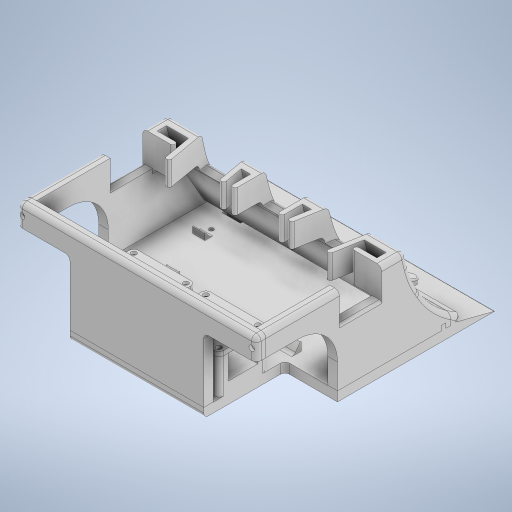
# Autodesk Inventor part: bodyv2
Saved by Autodesk Inventor 2024 (Build 280153000, 153)
## iProperties
Created: 2023-10-20
Part Number: bodyv2
Material: Generic
Document SubType Name: Modeling
Designer: kdcao
Density: 1 g/cm^3
Appearance: Default
Mass: 95.0467 g
Surface Area: 549.579 cm^2
Volume: 95.0467 cm^3
Author: kdcao
Autodesk Inventor part; units mm, degrees
ref_plane "YZ Plane" through (0, 0, 0) normal (1, 0, 0) x (0, 1, 0)
ref_plane "XZ Plane" through (0, 0, 0) normal (0, 1, 0) x (-1, 0, 0)
ref_plane "XY Plane" through (0, 0, 0) normal (0, 0, 1) x (1, 0, 0)
sketch "Sketch1" plane through (0, 0, 0) normal (0, 1, 0) x (-1, 0, 0)
  line L0 (-50, 50) -> (50, 50)
  line L1 (50, 50) -> (50, -50)
  line L2 (50, -50) -> (-50, -50)
  line L3 (-50, -50) -> (-50, 50)
  line L4 (-50, 50) -> (50, -50) construction
  line L5 (50, 50) -> (-50, -50) construction
  point P0 (0, 0)
  dimension "d0" = 100
  dimension "d1" = 100
  constraints: 12 end point, 2 midpoint, 2 parallel, 1 horizontal, 1 perpendicular
  measures "d0" distance of L0.end L1.end
  measures "d1" distance of L1.end L2.end
extrude "Extrusion1" add sketch "Sketch1" along normal blind 40
sketch "Sketch2" plane through (50, 0, 50) normal (1, 0, 0) x (0, 0, -1)
  line L0 (100, 0) -> (100, 40) projected
  line L1 (100, 0.1) -> (76.9136, 8.5028)
  line L2 (76.9136, 8.5028) -> (65.3666, 28.5028)
  line L3 (100, 40) -> (0, 40) projected
  line L4 (100, 40) -> (100, 0.1)
  line L5 (0, 0) -> (100, 0) projected
  line L6 (62.5, 40) -> (65.3666, 28.5028)
  point P0 (50, 0)
  dimension "d4" = 20
  dimension "d5" = 60
  dimension "d6" = 0.1
  dimension "d18" = 62.5
  dimension "d19" = 76
  dimension "d20" = 20
  constraints: 8 end point, 2 point on line, 1 vertical
  measures "d4" angle of L5 L1
  measures "d5" angle of L3 L2
  measures "d6" distance of L0.start L1.start
  measures "d18" distance of L6.start L3.end
  measures "d19" angle of L6 L3
  measures "d20" vertical distance of L1.end L2.end
extrude "Extrusion2" cut sketch "Sketch2" against normal through all
shell "Shell1" thickness 4 removed faces 1 at (16.6667, 40, 29.1667)
sketch "Sketch3" plane through (50, 0, 50) normal (1, 0, 0) x (0, 0, -1)
  circle A0 centre (17.5, 14.5) radius 16.5
  line L0 (0, 0) -> (0, 40) projected
  line L1 (0, 0) -> (100, 0) projected
  line L2 (0, 14.5) -> (0, 0)
  line L3 (0, 0) -> (34, 0)
  line L4 (34, 14.5) -> (34, 0)
  line L5 (17.5, 31) -> (0, 31)
  line L6 (91.2716, 1.5875) -> (0, 1.5875)
  point P0 (50, 0)
  dimension "d12" = 33
  dimension "d13" = 17.5
  dimension "d14" = 14.5
  dimension "d229" = 34
  dimension "d230" = 90
  dimension "d231" = 1.5875
  constraints: 10 end point, 3 point on line, 2 perpendicular, 2 point on circle, 1 centre point, 1 collinear, 1 tangent
  measures "d12" diameter of A0
  measures "d13" distance from line of L0 A0.centre
  measures "d14" distance from line of L1 A0.centre
  measures "d229" distance from line of L0.start L4
  measures "d230" angle of L6 L4
  measures "d231" distance from line of L1 L6.start
extrude "Extrusion3" cut sketch "Sketch3" against normal blind 22 contours A0 L6 | L4 L6 A0 | A0 L6 L0 L5 | L6 L4 L1 A0 | A0 L1 L6 | A0 L1 L0 L6
ref_plane "Work Plane1" through (0, 0, -50) normal (1, 0, 0) x (0, 0, -1)
mirror "Mirror1" about plane through (0, 0, -50) normal (1, 0, 0) of "Extrusion3"
fillet "Fillet1" radius 43.275 1 edges at (0, 8.5028, -26.9136)
fillet "Fillet2" radius 40 1 edges at (0, 28.5028, -15.3666)
sketch "Sketch27" plane through (-50, 40, 50) normal (0, 0, 1) x (1, 0, 0)
  line L0 (0, -9) -> (0, 0) projected
  line L1 (100, -9) -> (100, 0) projected
  point P0 (50, -40)
  point P1 (2, -4.5)
  point P2 (98, -4.5)
  point P3 (0, -4.5)
  point P4 (100, -4.5)
  dimension "d156" = 2
  dimension "d157" = 0
  dimension "d158" = 2
  dimension "d159" = 0
  constraints: 2 midpoint
  measures "d156" distance from line of L0 point (2, -4.5)
  measures "d157" vertical distance of point (0, -4.5) point (2, -4.5)
  measures "d158" distance from line of L1 point (98, -4.5)
  measures "d159" vertical distance of point (100, -4.5) point (98, -4.5)
hole "Hole5" at (-48, 35.5, 50) at (48, 35.5, 50) direction (0, 0, -1) diameter 1.75 depth 5.83 counterbore diameter 2.2 counterbore depth 1.2
sketch "Sketch28" plane through (0, 0, 0) normal (0, -1, 0) x (1, 0, 0)
  line L0 (-28, 50) -> (28, 50) projected
  line L1 (28, 16) -> (28, 50) projected
  line L2 (-28, 50) -> (-28, 16) projected
  line L3 (-50, -50) -> (-50, 16) projected
  line L4 (-28, 16) -> (-50, 16) projected
  line L5 (50, 16) -> (28, 16) projected
  line L6 (50, 16) -> (50, -50) projected
  point P0 (0, 0)
  point P1 (-24, 48)
  point P2 (24, 48)
  point P3 (-48, 12)
  point P4 (48, 12)
  dimension "d160" = 2
  dimension "d161" = 2
  dimension "d162" = 4
  dimension "d163" = 4
  dimension "d164" = 2
  dimension "d165" = 4
  dimension "d166" = 4
  dimension "d167" = 2
  measures "d160" distance from line of L0 point (-24, 48)
  measures "d161" distance from line of L0 point (24, 48)
  measures "d162" distance from line of L1 point (24, 48)
  measures "d163" distance from line of L2 point (-24, 48)
  measures "d164" distance from line of L3 point (-48, 12)
  measures "d165" distance from line of L4 point (-48, 12)
  measures "d166" distance from line of L5 point (48, 12)
  measures "d167" distance from line of L6 point (48, 12)
hole "Hole6" at (-24, 0, 48) at (24, 0, 48) at (-48, 0, 12) at (48, 0, 12) direction (0, 1, 0) diameter 1.75 depth 5.83 counterbore diameter 2.2 counterbore depth 1.2
sketch "Sketch4" plane through (50, 40, 50) normal (1, 0, 0) x (0, 0, -1)
  line L0 (-2.2168, -36) -> (77.4409, -36)
  arc A0 (69.0382, -17.8566) -> (91.7145, -36.8843) centre (106.5154, 3.7809) ccw projected
  line L1 (34, -40) -> (100, -40) projected
  line L2 (77.4409, -36) -> (77.4409, -34)
  line L3 (77.4409, -34) -> (79.4409, -34)
  line L4 (79.4409, -36) -> (81.4409, -36)
  line L5 (78.6988, -29.3469) -> (78.6988, -29.3697)
  line L6 (79.4409, -34) -> (79.4409, -36)
  line L7 (81.4409, -36) -> (81.4409, -31.4894)
  line L8 (0, -40) -> (0, -9) projected
  point P0 (50, -40)
  point P1 (78.6988, -29.3697)
  dimension "d73" = 2
  dimension "d75" = 4
  dimension "d76" = 2
  dimension "d77" = 2
  dimension "d78" = 2
  dimension "d79" = 81.4409
  constraints: 14 end point, 3 perpendicular, 3 point on circle, 2 vertical, 1 horizontal
  measures "d73" distance of L2.end L3.end
  measures "d75" distance between parallel lines of L1 L0
  measures "d76" distance of L0.end L2.end
  measures "d77" distance of L3.end L4.start
  measures "d78" distance of L4.start L4.end
  measures "d79" distance from line of L8 L4.end
split body "Split1" sketch "Sketch4" result two bodies curves L0 L2 L3 L6 L4 L7 first body at (9.3333, 22, 49.5)
sketch "Sketch5" plane through (-50, 0, -50) normal (-1, 0, 0) x (0, 0, 1)
  line L0 (66, 4) -> (22.5591, 4) projected
  line L1 (39.2, 4) -> (39.2, 7)
  line L2 (39.2, 7) -> (36.8561, 4)
  line L3 (36.8561, 4) -> (39.2, 4)
  line L4 (100, 4) -> (100, 0) projected
  line L5 (66, 0) -> (66, 4) projected
  point P0 (50, 0)
  point P1 (17.4103, 4)
  dimension "d28" = 3
  dimension "d29" = 38
  dimension "d43" = 26.8
  constraints: 6 end point, 2 perpendicular, 1 point on line
  measures "d28" distance of L1.start L1.end
  measures "d29" angle of L1 L2
  measures "d43" distance from line of L1.start L5
ref_plane "Work Plane2" through (-37.5, 0, -50) normal (-1, 0, 0) x (0, 0, 1)
extrude "Extrusion4" add sketch "Sketch5" against normal blind 5.15 from surface at -12.5 bodies 3
sketch "Sketch6" plane through (-28, 0, 16) normal (-1, 0, 0) x (0, 0, 1)
  line L0 (34, 4) -> (0, 4) projected
  line L1 (7.3, 4) -> (7.3, 18.6)
  line L2 (7.3, 18.6) -> (11.3, 18.6)
  line L3 (11.3, 18.6) -> (11.3, 8.5)
  line L4 (11.3, 8.5) -> (23.7, 8.5)
  line L5 (23.7, 8.5) -> (23.7, 18.6)
  line L6 (23.7, 18.6) -> (27.7, 18.6)
  line L7 (27.7, 18.6) -> (27.7, 4)
  line L8 (7.3, 4) -> (27.7, 4)
  line L9 (34, 4) -> (34, 0) projected
  line L10 (7.3, 18.6) -> (27.7, 18.6)
  line L11 (27.7, 18.6) -> (27.7, 20.6)
  line L12 (27.7, 20.6) -> (7.3, 20.6)
  line L13 (7.3, 20.6) -> (7.3, 18.6)
  point P0 (-16, 0)
  point P1 (27.7, 18.6)
  dimension "d34" = 12.4
  dimension "d38" = 4
  dimension "d39" = 4
  dimension "d40" = 10.3
  dimension "d168" = 10.1
  dimension "d169" = 14.6
  dimension "d170" = 2
  dimension "d171" = 20.4
  constraints: 24 end point, 7 perpendicular, 4 point on line, 2 parallel, 1 collinear, 1 horizontal
  measures "d34" distance of L3.end L4.end
  measures "d38" distance of L5.end L6.end
  measures "d39" distance of L1.end L2.end
  measures "d40" distance between parallel lines of L9 L5
  measures "d168" distance of L2.end L3.end
  measures "d169" distance of L6.end L7.end
  measures "d170" distance of L12.end L1.end
  measures "d171" distance of L11.end L12.end
extrude "Extrusion5" add sketch "Sketch6" against normal blind 25.7875 contours L0 L1 L2 L3 L4 L5 L6 L7 | L6 L10 L2 L13 L12 L11 bodies 3
mirror "Mirror2" about plane through (0, 0, -50) normal (1, 0, 0) of "Extrusion5", "Extrusion4" bodies 3
sketch "Sketch7" plane through (-28, 0, 16) normal (-1, 0, 0) x (0, 0, 1)
  line L0 (-6.8, 4) -> (-6.8, 8)
  line L1 (-6.8, 8) -> (-3.8, 4)
  line L2 (-26.8, 7) -> (-26.8, 4) projected
  line L3 (-6.8, 4) -> (-3.8, 4)
  point P0 (-16, 0)
  point P1 (0, 4)
  dimension "d45" = 3
  dimension "d46" = 4
  dimension "d232" = 20
  constraints: 6 end point, 1 horizontal, 1 point on line
  measures "d45" distance from line of L1.end L0
  measures "d46" distance of L0.start L0.end
  measures "d232" distance between parallel lines of L0 L2
extrude "Extrusion6" add sketch "Sketch7" against normal blind 5.15 bodies 3
mirror "Mirror3" about plane through (0, 0, -50) normal (1, 0, 0) of "Extrusion6" bodies 3
sketch "Sketch9" plane through (28, 4, 16) normal (0, 1, 0) x (1, 0, 0)
  line L0 (-66.85, 42.8) -> (-59.15, 42.8)
  line L1 (-59.15, 42.8) -> (-59.15, 30)
  line L2 (-59.15, 30) -> (-66.85, 30)
  line L3 (-66.85, 30) -> (-66.85, 42.8)
  line L4 (-66.85, 42.8) -> (-59.15, 30) construction
  line L5 (-59.15, 42.8) -> (-66.85, 30) construction
  line L6 (-78, 0) -> (-78, 43.4409) projected
  line L7 (-78, 0) -> (-56, 0) projected
  point P0 (-28, 16)
  point P1 (-63, 36.4)
  point P2 (-78, 48.5897)
  point P3 (-63, 30)
  dimension "d49" = 12.8
  dimension "d50" = 7.7
  dimension "d51" = 15
  dimension "d52" = 30
  constraints: 12 end point, 3 midpoint, 2 parallel, 1 horizontal, 1 perpendicular
  measures "d49" distance of L2.end L0.start
  measures "d50" distance of L1.end L2.end
  measures "d51" distance from line of L6 point (-63, 30)
  measures "d52" distance between parallel lines of L7 L2
extrude "Extrusion7" cut sketch "Sketch9" along normal blind 3 from surface at -4 bodies 3
mirror "Mirror4" about plane through (0, 0, -50) normal (1, 0, 0) of "Extrusion7" bodies 3
ref_plane "Work Plane4" through (-50, 40, -10.5) normal (0, 0, 1) x (1, 0, 0)
sketch "Sketch12" plane through (-50, 40, -10.5) normal (0, 0, 1) x (1, 0, 0)
  line L0 (50.0586, -12.0127) -> (41.2086, -12.0127)
  line L1 (41.2086, -12.0127) -> (41.2086, 0.5873)
  line L2 (41.2086, 0.5873) -> (58.9086, 0.5873)
  line L3 (58.9086, 0.5873) -> (58.9086, -12.0127)
  line L4 (58.9086, -12.0127) -> (50.0586, -12.0127)
  point P0 (50, -40)
  dimension "d61" = 12.6
  dimension "d62" = 17.7
  constraints: 10 end point, 4 perpendicular, 1 collinear, 1 horizontal, 1 point on line
  measures "d61" distance of L2.end L3.end
  measures "d62" distance of L1.end L2.end
extrude "Extrusion9" cut sketch "Sketch12" along normal mid plane 14.7625 bodies 2
ref_plane "Work Plane5" through (34.4281, 50.6, -7.4264) normal (0.1736482, 0, -0.9848078) x (0, -1, 0)
sketch "Sketch13" plane through (34.4281, 50.6, -7.4264) normal (0.1736482, 0, -0.9848078) x (0, -1, 0)
  line L0 (10.6, -0.1431) -> (23.2, -0.1431)
  line L1 (23.2, -0.1431) -> (23.2, 17.5569)
  line L2 (23.2, 17.5569) -> (10.6, 17.5569)
  line L3 (10.6, 17.5569) -> (10.6, -0.1431)
  line L4 (10.6, 25.2969) -> (10.6, -11.231) projected
  line L5 (10.6, 25.2969) -> (22.6127, 25.817) projected
  point P0 (50.6, 32.6154)
  point P1 (16.6063, 25.5569)
  dimension "d65" = 17.7
  dimension "d66" = 12.6
  dimension "d263" = 8
  constraints: 8 end point, 2 parallel, 1 horizontal, 1 midpoint, 1 perpendicular, 1 point on line
  measures "d65" distance of L2.end L0.start
  measures "d66" distance of L1.end L2.end
  measures "d263" distance from line of point (16.606, 25.557) L2
extrude "Extrusion10" cut sketch "Sketch13" along normal mid plane 20 bodies 2
ref_plane "Work Plane6" through (-34.4281, 38, -7.4264) normal (0.1736482, 0, 0.9848078) x (0, 1, 0)
sketch "Sketch14" plane through (-34.4281, 38, -7.4264) normal (0.1736482, 0, 0.9848078) x (0, 1, 0)
  line L0 (-10.6, -0.8394) -> (2, -0.8394)
  line L1 (2, -0.8394) -> (2, -17.4394)
  line L2 (2, -17.4394) -> (-10.6, -17.4394)
  line L3 (-10.6, -17.4394) -> (-10.6, -0.8394)
  line L4 (2, 11.231) -> (2, -25.4124) projected
  line L5 (-10.0127, -25.9325) -> (2, -25.4124) projected
  point P0 (-38, -32.6154)
  point P1 (-4.0063, -25.6724)
  dimension "d69" = 16.6
  dimension "d70" = 12.6
  constraints: 8 end point, 2 parallel, 1 horizontal, 1 midpoint, 1 perpendicular, 1 point on line
  measures "d69" distance of L0.end L1.end
  measures "d70" distance of L1.end L2.end
extrude "Extrusion11" cut sketch "Sketch14" along normal mid plane 20 bodies 2
sketch "Sketch15" plane through (0, 0, 0) normal (0, -1, 0) x (1, 0, 0)
  line L0 (31.15, -26.8) -> (31.15, -14) projected
  line L1 (38.85, -26.8) -> (31.15, -26.8) projected
  line L2 (31.15, -24.5) -> (38.85, -24.5)
  line L3 (38.85, -24.5) -> (38.85, -26.8)
  line L4 (38.85, -26.8) -> (31.15, -26.8)
  line L5 (31.15, -26.8) -> (31.15, -24.5)
  circle A0 centre (35, -16.1508) radius 0.875
  line L6 (50, 16) -> (50, -50) projected
  line L7 (50, -50) -> (-50, -50) projected
  point P0 (0, 0)
  dimension "d80" = 15
  dimension "d81" = 1.75
  dimension "d82" = 2.3
  dimension "d83" = 33.8492
  constraints: 8 end point, 2 parallel, 1 centre point, 1 horizontal, 1 perpendicular, 1 point on line
  measures "d80" distance from line of L6 A0.centre
  measures "d81" diameter of A0
  measures "d82" distance of L2.end L1.start
  measures "d83" distance from line of L7 A0.centre
extrude "Extrusion12" cut sketch "Sketch15" against normal through all bodies 3
mirror "Mirror5" about plane through (0, 0, -50) normal (1, 0, 0) of "Extrusion12" bodies 3
sketch "Sketch16" plane through (50, 40, 50) normal (1, 0, 0) x (0, 0, -1)
  line L0 (4, -20.7805) -> (4, 0)
  line L1 (0, -9) -> (0, 0) projected
  point P0 (50, -40)
  dimension "d86" = 4
  constraints: 2 end point
  measures "d86" distance between parallel lines of L1 L0
split body "Split2" sketch "Sketch16" result two bodies bodies 2 curves L0 first body at (9.3333, 22, 49.5)
sketch "Sketch17" plane through (0, 40, 0) normal (0, 1, 0) x (1, 0, 0)
  line L0 (35.4679, 12.5) -> (32.6467, -3.5)
  line L1 (32.6467, -3.5) -> (34.6467, -3.8527)
  line L2 (34.6467, -3.8527) -> (37.4679, 12.1473)
  line L3 (37.4679, 12.1473) -> (35.4679, 12.5)
  line L4 (17.4949, 12.5) -> (15.2026, -0.5)
  line L5 (15.2026, -0.5) -> (13.2026, -0.1473)
  line L6 (13.2026, -0.1473) -> (15.4327, 12.5)
  line L7 (16.768, 8.3776) -> (17.4949, 12.5) projected
  line L8 (17.4949, 12.5) -> (8.9086, 12.5) projected
  line L9 (15.4327, 12.5) -> (17.4949, 12.5)
  point P0 (0, 0)
  point P1 (17.1314, 10.4388)
  point P2 (14.2026, -0.3237)
  dimension "d87" = 2
  dimension "d88" = 16
  dimension "d89" = 2
  dimension "d264" = 17.7
  dimension "d266" = 13
  constraints: 16 end point, 4 parallel, 2 midpoint, 2 perpendicular, 1 horizontal
  measures "d87" horizontal distance of L0.end L1.end
  measures "d88" vertical distance of L1.end L2.end
  measures "d89" horizontal distance of L4.end L5.end
  measures "d264" distance from line of point (17.131, 10.439) L0
  measures "d266" vertical distance of L4.start L4.end
extrude "Extrusion13" add sketch "Sketch17" against normal blind 10 bodies 5
mirror "Mirror6" about plane through (0, 0, -50) normal (1, 0, 0) of "Extrusion13" bodies 5
sketch "Sketch18" plane through (0, 40, 0) normal (0, 1, 0) x (1, 0, 0)
  line L0 (17.4949, 12.5) -> (8.9086, 12.5) projected
  line L1 (8.9086, 12.5) -> (8.9086, 0)
  line L2 (8.9086, 0) -> (10.9086, 0)
  line L3 (10.9086, 0) -> (10.9086, 12.5)
  line L4 (10.9086, 12.5) -> (8.9086, 12.5)
  line L5 (-8.7914, 16.0057) -> (-8.7914, 11.3726) projected
  line L6 (-8.7914, 12.5) -> (-8.7914, 0)
  line L7 (-8.7914, 0) -> (-10.7914, 0)
  line L8 (-10.7914, 0) -> (-10.7914, 12.5)
  line L9 (-10.7914, 12.5) -> (-8.7914, 12.5)
  point P0 (0, 0)
  point P1 (-8.7914, 15.4951)
  point P2 (-8.7914, 11.3726)
  dimension "d94" = 2
  dimension "d95" = 2
  dimension "d96" = 12.5
  constraints: 16 end point, 4 parallel, 3 perpendicular, 3 point on line, 1 collinear
  measures "d94" distance of L1.end L2.end
  measures "d95" distance of L6.end L7.end
  measures "d96" distance of L2.end L3.end
extrude "Extrusion14" add sketch "Sketch18" against normal blind 10 bodies 5
sketch "Sketch31" plane through (-28, 20.6, 43.7) normal (0, 1, 0) x (1, 0, 0)
  line L0 (0, 20.4) -> (25.7875, 20.4) projected
  line L1 (25.7875, 20.4) -> (25.7875, 0) projected
  line L2 (0, 0) -> (25.7875, 0) projected
  line L3 (0, 0) -> (0, 20.4) projected
  point P0 (28, 43.7)
  point P1 (23.7875, 18.4)
  point P2 (23.7875, 2)
  point P3 (2, 2)
  point P4 (2, 18.4)
  dimension "d180" = 2
  dimension "d181" = 2
  dimension "d182" = 2
  dimension "d183" = 2
  dimension "d184" = 2
  dimension "d185" = 2
  dimension "d186" = 2
  dimension "d187" = 2
  measures "d180" distance from line of L0 point (23.787, 18.4)
  measures "d181" distance from line of L1 point (23.787, 18.4)
  measures "d182" distance from line of L1 point (23.787, 2)
  measures "d183" distance from line of L2 point (23.787, 2)
  measures "d184" distance from line of L2 point (2, 2)
  measures "d185" distance from line of L3 point (2, 2)
  measures "d186" distance from line of L0 point (2, 18.4)
  measures "d187" distance from line of L3 point (2, 18.4)
hole "Hole7" at (-4.2125, 20.6, 25.3) at (-4.2125, 20.6, 41.7) at (-26, 20.6, 41.7) at (-26, 20.6, 25.3) direction (0, -1, 0) diameter 1.75 depth 5.83 counterbore diameter 2.2 counterbore depth 1.2 bodies 3
mirror "Mirror7" about plane through (0, 0, -50) normal (1, 0, 0) of "Hole7" bodies 3
sketch "Sketch32" plane through (-28, 0, 16) normal (-1, 0, 0) x (0, 0, 1)
  line L0 (7.3, 4) -> (7.3, 20.6) projected
  line L1 (7.3, 18.6) -> (27.7, 18.6)
  line L2 (27.7, 20.6) -> (27.7, 4) projected
  point P0 (-16, 0)
  point P1 (11.3, 18.6)
  constraints: 3 point on line, 2 end point, 1 horizontal
split body "Split6" sketch "Sketch32" result two bodies bodies 3 curves L1 first body at (11.7768, 20.1, 36.025) (-11.7768, 20.1, 36.025)
fillet "Fillet4" radius 2 8 edges at (-28, 19.6, 43.7) (-28, 19.6, 23.3) (-2.2125, 19.6, 23.3) (-2.2125, 19.6, 43.7) (-28, 11.3, 43.7) (-28, 11.3, 23.3) (-2.2125, 11.3, 23.3) (-2.2125, 11.3, 43.7)
mirror "Mirror8" about plane through (0, 0, -50) normal (1, 0, 0) of "Fillet4"
sketch "Sketch34" plane through (0, 40, 0) normal (0, 1, 0) x (1, 0, 0)
  line L0 (-46, -46) -> (-46, 8.3776) projected
  line L1 (-50, -32.5) -> (-50, -16) projected
  line L2 (-46, 2.5) -> (-50, 2.5)
  line L3 (-50, 2.5) -> (-50, -15.2)
  line L4 (-50, -15.2) -> (-46, -15.2)
  line L5 (-46, -15.2) -> (-46, 2.5)
  line L6 (-34.4703, 12.5) -> (-50, 12.5) projected
  point P0 (0, 0)
  point P1 (-46, -15.2)
  dimension "d196" = 17.7
  dimension "d197" = 10
  constraints: 8 end point, 2 parallel, 2 point on line, 1 horizontal, 1 perpendicular
  measures "d196" distance of L2.end L3.end
  measures "d197" distance between parallel lines of L6 L2
extrude "Extrusion15" cut sketch "Sketch34" against normal blind 12.6 bodies 5
sketch "Sketch35" plane through (0, 40, 0) normal (0, 1, 0) x (1, 0, 0)
  line L0 (-50, 12.5) -> (-50, 2.5) projected
  line L1 (-50, 2.5) -> (-37.5, 2.5)
  line L2 (-37.5, 2.5) -> (-37.5, 4.5)
  line L3 (-37.5, 4.5) -> (-50, 4.5)
  line L4 (-50, 4.5) -> (-50, 2.5)
  point P0 (0, 0)
  dimension "d200" = 12.5
  dimension "d201" = 2
  constraints: 8 end point, 2 parallel, 1 horizontal, 1 perpendicular
  measures "d200" distance of L2.end L3.end
  measures "d201" distance of L1.end L2.end
extrude "Extrusion16" add sketch "Sketch35" against normal blind 12.6 bodies 5
mirror "Mirror9" about plane through (0, 0, -50) normal (1, 0, 0) of "Extrusion15", "Extrusion16" bodies 5
fillet "Fillet8" radius 2 26 edges at (50, 40, 48) (0, 40, 50) (-50, 40, 48) (50, 35.5, 50) (-50, 35.5, 50) (-28, 31, 48) (28, 31, 48) (50, 40, -7.5) (42.734, 40, -12.5) (50, 40, 30.6) (-50, 40, 30.6) (-50, 40, -7.5) (-42.2351, 40, -12.5) (-13.2028, 40, -12.5) (13.2018, 40, -12.5) (50, 22.8888, -18.6078) (50, 14.659, -24.5054) (50, 36.9787, -13.2533) (50, 28.65, -15.7311) (-50, 22.8888, -18.6078) (-50, 28.65, -15.7311) (-50, 36.9787, -13.2533) (-50, 14.659, -24.5054) (0, 0, 50) (28, 2, 16) (-28, 2, 16)
fillet "Fillet9" radius 1 18 edges at (-50, 27.4, 6.35) (50, 27.4, 6.35) (37.5, 33.7, -4.5) (37.5, 33.7, -2.5) (32.6467, 35, 3.5) (34.6467, 35, 3.8527) (13.2026, 35, 0.1473) (15.2026, 35, 0.5) (10.9086, 35, 0) (8.9086, 35, 0) (-8.7914, 35, 0) (-10.7914, 35, 0) (-15.2026, 35, 0.5) (-13.2026, 35, 0.1473) (-32.6467, 35, 3.5) (-34.6467, 35, 3.8527) (-37.5, 33.7, -4.5) (-37.5, 33.7, -2.5)
sketch "Sketch36" plane through (-50, 0, -50) normal (-1, 0, 0) x (0, 0, 1)
  arc A0 (8.2855, 3.1157) -> (18.5591, 8.5106) centre (-6.5154, 43.7809) ccw projected
  line L0 (18.5591, 4) -> (18.5591, 8.5106) projected
  line L1 (0, 0) -> (66, 0) projected
  line L2 (0.15, 0) -> (14.55, 3.6975)
  line L3 (14.55, 3.6975) -> (14.0365, 5.6975)
  line L4 (14.0365, 5.6975) -> (-1.9913, 0)
  line L5 (-1.9913, 0) -> (0.15, 0)
  line L6 (0.2518, 0.0261) -> (0.4, 0)
  line L7 (0.15, 0) -> (0.4, 0)
  point P0 (50, 0)
  dimension "d210" = 2
  dimension "d211" = 0.15
  dimension "d213" = 14.4
  dimension "d214" = 17.0103
  dimension "d226" = 0.25
  dimension "d227" = 10
  constraints: 12 end point, 4 point on line, 1 collinear, 1 horizontal, 1 perpendicular, 1 point on circle
  measures "d210" vertical distance of L2.end L3.end
  measures "d211" distance of L1.start L2.start
  measures "d213" horizontal distance of L2.end L2.start
  measures "d214" distance of L3.end L4.end
  measures "d226" distance of L2.start L6.end
  measures "d227" angle of L1 L6
extrude "Extrusion17" cut sketch "Sketch36" against normal through all bodies 7
sketch "Sketch37" plane through (-50, 0, -49.85) normal (0, 0.9685803, -0.2487012) x (1, 0, 0)
  circle A0 centre (26, -10.1171) radius 2.5
  line L0 (0, -14.8671) -> (0, -0.1051) projected
  line L1 (100, -14.8671) -> (0, -14.8671) projected
  point P0 (50, -48.2837)
  point P1 (0, 0)
  dimension "d217" = 5
  dimension "d218" = 26
  dimension "d219" = 4.75
  constraints: 1 centre point
  measures "d217" diameter of A0
  measures "d218" distance from line of L0 A0.centre
  measures "d219" distance from line of L1 A0.centre
extrude "Extrusion18" add sketch "Sketch37" along normal blind 2 bodies 7
fillet "Fillet10" radius 0.5 1 edges at (-26.5, 4.4533, -40.5482)
mirror "Mirror10" about plane through (0, 0, -50) normal (1, 0, 0) of "Extrusion18", "Fillet10" bodies 7
fillet "Fillet11" radius 0.5 1 edges at (0, 5.6975, -35.9635)
fillet "Fillet13" radius 2 6 edges at (50, 5.6432, -35.8415) (50, 4.509, -35.6584) (50, 7.1369, -33.4949) (-50, 5.6432, -35.8415) (-50, 4.509, -35.6584) (-50, 7.1369, -33.4949)
fillet "Fillet14" radius 2 4 edges at (-25.425, 4, 12.2) (25.425, 4, 12.2) (-34.925, 4, -13.1439) (34.925, 4, -13.1439)
fillet "Fillet15" radius 0.2 4 edges at (34.925, 7, -10.8) (25.425, 8, 9.2) (-25.425, 8, 9.2) (-34.925, 7, -10.8)
sketch "Sketch38" plane through (28, 4, 46) normal (0, 0, -1) x (-1, 0, 0)
  line L0 (21.75, 24) -> (25.75, 24)
  line L1 (25.75, 24) -> (25.75, 28)
  line L2 (25.75, 28) -> (21.75, 28)
  line L3 (21.75, 28) -> (21.75, 24)
  line L4 (21.75, 24) -> (25.75, 28) construction
  line L5 (25.75, 24) -> (21.75, 28) construction
  line L6 (31.75, 24) -> (35.75, 24)
  line L7 (35.75, 24) -> (35.75, 28)
  line L8 (35.75, 28) -> (31.75, 28)
  line L9 (31.75, 28) -> (31.75, 24)
  line L10 (31.75, 24) -> (35.75, 28) construction
  line L11 (35.75, 24) -> (31.75, 28) construction
  line L12 (-22, 27) -> (-2, 27) projected
  line L13 (76, 36) -> (-20, 36) projected
  point P0 (28, -4)
  point P1 (23.75, 26)
  point P2 (33.75, 26)
  point P3 (28, 36)
  point P4 (28, 36)
  point P5 (28, 36)
  dimension "d235" = 4
  dimension "d236" = 4
  dimension "d237" = 4
  dimension "d238" = 4
  dimension "d239" = 1
  dimension "d241" = 4.25
  dimension "d242" = 5.75
  constraints: 24 end point, 7 midpoint, 4 parallel, 2 horizontal, 2 perpendicular, 1 point on line
  measures "d235" distance of L1.end L2.end
  measures "d236" distance of L7.end L8.end
  measures "d237" distance of L2.end L0.start
  measures "d238" distance of L8.end L6.start
  measures "d239" distance between parallel lines of L12 L2
  measures "d241" horizontal distance of point (28, 36) point (23.75, 26)
  measures "d242" horizontal distance of point (33.75, 26) point (28, 36)
extrude "Extrusion19" add sketch "Sketch38" along normal blind 6.5 bodies 4
sketch "Sketch39" plane through (2.25, 32, 46) normal (0, 1, 0) x (1, 0, 0)
  line L0 (0, 0) -> (0, 6.5) projected
  line L1 (-10, 0) -> (-10, 6.5) projected
  line L2 (-10, 6.5) -> (-6, 6.5) projected
  line L3 (-50.25, 0) -> (45.75, 0) projected
  point P0 (-2.25, 46)
  point P1 (2, 4.5)
  point P2 (-8, 4.5)
  dimension "d252" = 2
  dimension "d253" = 2
  dimension "d255" = 4.5
  dimension "d256" = 4.5
  measures "d252" distance from line of L0 point (2, 4.5)
  measures "d253" distance from line of L1 point (-8, 4.5)
  measures "d255" distance from line of L3 point (2, 4.5)
  measures "d256" distance from line of L3 point (-8, 4.5)
hole "Hole8" at (4.25, 32, 41.5) at (-5.75, 32, 41.5) direction (0, -1, 0) diameter 1.75 end through all bodies 4
fillet "Fillet16" radius 2 8 edges at (2.25, 30, 39.5) (6.25, 30, 39.5) (2.25, 30, 46) (-7.75, 30, 39.5) (-3.75, 30, 39.5) (-7.75, 30, 46) (-3.75, 30, 46) (6.25, 30, 46)
sketch "Sketch40" plane through (-50, 0, 16) normal (-1, 0, 0) x (0, 0, 1)
  line L0 (-43.4409, 6) -> (-45.4409, 6) projected
  line L1 (-45.3909, 6) -> (-45.4409, 6)
  line L2 (-45.4409, 6) -> (-45.4409, 4)
  line L3 (-45.4409, 4) -> (-45.3909, 4)
  line L4 (-45.3909, 4) -> (-45.3909, 6)
  point P0 (-16, 0)
  dimension "d258" = 0.05
  constraints: 8 end point, 2 parallel, 1 horizontal, 1 perpendicular, 1 point on line
  measures "d258" distance of L2.end L3.end
extrude "Extrusion20" cut sketch "Sketch40" against normal through all bodies 7
mirror "Mirror11" about plane through (0, 0, -50) normal (1, 0, 0) of "Extrusion10" bodies 5
fillet "Fillet17" radius 2 11 edges at (27.1446, 27.4, -16.261) (36.2118, 30, -10.8708) (9.9086, 30, -10.8708) (16.1765, 30, -10.8708) (0.0586, 27.9873, -16.0057) (-9.7914, 30, -10.8708) (-16.1765, 30, -10.8708) (-27.1446, 27.4, -16.261) (-36.2118, 30, -10.8708) (-46, 27.4, -3.5) (46, 27.4, -3.5)
body "Solid4"
body "Solid5"
body "Solid12"
body "Solid13"
